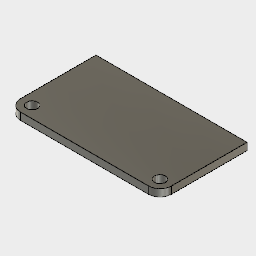
1982 MPR121 (Autodesk Fusion 360 design; units mm, degrees)
Autodesk Fusion 360 part; units mm, degrees
sketch "Sketch1" plane through (0, 0, 0) normal (0, 0, 1) x (1, 0, 0)
  line L0 (0, 0) -> (33.02, 0)
  line L1 (33.02, 0) -> (33.02, 19.05)
  line L2 (33.02, 19.05) -> (0, 19.05)
  line L3 (0, 19.05) -> (0, 0)
  circle A0 centre (30.48, 2.54) radius 1.205
  line L4 (16.51, 19.05) -> (16.51, 0) construction
  line L5 (0, 9.525) -> (33.02, 9.525) construction
  circle A1 centre (2.54, 2.54) radius 1.205
  dimension "d1" = 33.02
  dimension "d2" = 19.05
  dimension "d3" = 2.41
  dimension "d4" = 2.54
  dimension "d5" = 30.48
  measures "d1" distance of L0.start L0.end
  measures "d2" distance of L0.start L2.end
  measures "d3" diameter of A0
  measures "d4" distance of L0 A0.centre
  measures "d5" distance of L3 A0.centre
extrude "Extrude1" add sketch "Sketch1" along normal blind 1.6
fillet "Fillet1" radius 2.54 2 edges at (0, 0, 0.8) (33.02, 0, 0.8)
